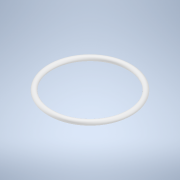
# Autodesk Inventor part: Уплотнительное кольцо
Saved by Autodesk Inventor 2021 (Build 250183000, 183)
## iProperties
Created: 2020-12-08
Part Number: Уплотнительное кольцо
Material: Алюминий 6061
Document SubType Name: Modeling
Designer: Тимоха
Mass: 23.5035 g
Surface Area: 58.0333 cm^2
Volume: 8.70499 cm^3
Density: 2.7 g/cm^3
Appearance: Алюминий — плоский
Author: Тимоха
Autodesk Inventor part; units mm, degrees
ref_plane "YZ Plane" through (0, 0, 0) normal (1, 0, 0) x (0, 1, 0)
ref_plane "XZ Plane" through (0, 0, 0) normal (0, 1, 0) x (-1, 0, 0)
ref_plane "XY Plane" through (0, 0, 0) normal (0, 0, 1) x (1, 0, 0)
sketch "Эскиз1" plane through (0, 0, 0) normal (0, 0, 1) x (1, 0, 0)
  line L0 (0, 0) -> (49, 0)
  circle A0 centre (49, 0) radius 3
  line L1 (0, 0) -> (0, 5.5778)
  dimension "d0" = 49
  dimension "d1" = 6
  constraints: 4 end point, 1 centre point, 1 coincident, 1 horizontal, 1 vertical
  measures "d0" distance of L0.start L0.end
  measures "d1" diameter of A0
revolve "Вращение1" add sketch "Эскиз1" angle 360 about axis through (0, 0, 0) along (0, 1, 0)
